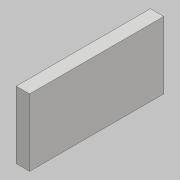
# Autodesk Inventor part: exercise3-7
Saved by Autodesk Inventor 2018 (Build 220112000, 112)
## iProperties
Created: 2020-09-23
Part Number: exercise3-7
Material: 一般
Document SubType Name: Modeling
Designer: 王鼎鈞
Density: 1 g/cm^3
Appearance: 預設
Author: 王鼎鈞
Autodesk Inventor part; units mm, degrees
ref_plane "YZ Plane" through (0, 0, 0) normal (1, 0, 0) x (0, 1, 0)
ref_plane "XZ Plane" through (0, 0, 0) normal (0, 1, 0) x (-1, 0, 0)
ref_plane "XY Plane" through (0, 0, 0) normal (0, 0, 1) x (1, 0, 0)
sketch "草圖1" plane through (0, 0, 0) normal (1, 0, 0) x (0, 1, 0)
  line L0 (-60, 30) -> (60, 30)
  line L1 (60, 30) -> (60, -30)
  line L2 (60, -30) -> (-60, -30)
  line L3 (-60, -30) -> (-60, 30)
  line L4 (-60, 30) -> (60, -30) construction
  line L5 (60, 30) -> (-60, -30) construction
  point P0 (0, 0)
  dimension "d0" = 120
  dimension "d1" = 60
  constraints: 12 end point, 2 midpoint, 2 parallel, 1 horizontal, 1 perpendicular
  measures "d0" distance of L1.end L2.end
  measures "d1" distance of L0.end L1.end
extrude "擠出1" add sketch "草圖1" along normal blind 12
